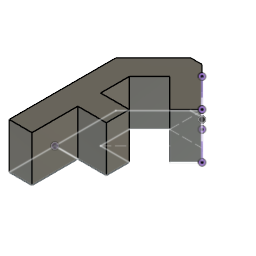
Phototransistor Mount (Autodesk Fusion 360 archive; units mm, degrees)
design "Lab Stand Mount"
Autodesk Fusion 360 part; units mm, degrees
sketch "Sketch1" plane through (0, 0, 0) normal (0, 0, 1) x (1, 0, 0) in component "Lab Stand Mount"
  line L0 (22.5, 0) -> (22.5, 10)
  line L1 (10, 0) -> (10, -20)
  line L2 (22.5, 10) -> (10, 10)
  line L3 (10, 22.5) -> (18.8388, 31.3388)
  line L4 (0, -20) -> (0, 0)
  line L5 (0, 0) -> (22.5, 0)
  line L6 (38.4099, 25.9099) -> (18.8388, 45.481)
  line L7 (10, 10) -> (10, 22.5)
  line L8 (0, 0) -> (10, 0)
  line L9 (31.3388, 18.8388) -> (38.4099, 25.9099)
  line L10 (18.8388, 31.3388) -> (32.981, 31.3388) construction
  line L11 (18.8388, 31.3388) -> (31.3388, 18.8388)
  line L12 (10, 10) -> (25.0888, 25.0888) construction
  line L13 (10, -20) -> (0, -20)
  line L14 (18.8388, 31.3388) -> (18.8388, 45.481) construction
  line L15 (18.8388, 45.481) -> (0, 26.6421)
  line L16 (0, 26.6421) -> (0, 0)
  line L17 (21.3388, 42.981) -> (16.3388, 42.981)
  dimension "d18" = 22.5
  dimension "d19" = 10
  dimension "d20" = 12.5
  dimension "d21" = 12.5
  dimension "d22" = 45
  dimension "d23" = 12.5
  dimension "d24" = 45
  dimension "d25" = 10
  dimension "d28" = 10
  dimension "d29" = 20
  dimension "d43" = 2.5
  constraint coincident L4.end L5.start
  constraint horizontal L5
  constraint perpendicular L0 L5
  constraint perpendicular L0 L2
  constraint perpendicular L2 L7
  constraint horizontal L10
  constraint midpoint L12.end L11
  constraint perpendicular L9 L11
  constraint perpendicular L6 L9
  constraint parallel L3 L12
  constraint horizontal L8
  constraint vertical L1
  constraint horizontal L13
  constraint vertical L4
  constraint perpendicular L10 L14
  constraint coincident L6.end L14
  constraint perpendicular L5 L16
  constraint coincident L6 L17.start
  constraint coincident L15 L17.end
  constraint perpendicular L14 L17
  constraint parallel L3 L15
  constraint coincident L10.end L6
  measures "d18" distance of L4.end L0.start
  measures "d19" distance of L0.end L0.start
  measures "d20" distance of L0.end L2.end
  measures "d21" distance of L2.end L3.start
  measures "d22" angle of L10 L11
  measures "d23" distance of L0.end L11
  measures "d24" angle of L2 L12
  measures "d25" distance of L6.start L9.start
  measures "d28" distance of L4.end L1.start
  measures "d29" distance of L4.start L4.end
  measures "d43" distance of L6.end L17
extrude "Extrude1" add sketch "Sketch1" along normal blind 20 contours L0 L2 L3 L5 L6 L7 L8 L9 L11 L15 L16 L17 | L1 L4 L5 L8 L13 in component "Lab Stand Mount"
sketch "Sketch2" plane through (32.1599, 32.1599, 0) normal (0.707107, 0.707107, 0) x (-0.707107, 0.707107, 0) in component "Lab Stand Mount"
  line L0 (0, 20) -> (0, 0) construction
  line L1 (8.8388, 10) -> (-8.8388, 10) construction
  line L2 (-3.25, 15.6292) -> (-6.5, 10)
  line L3 (-6.5, 10) -> (-3.25, 4.3708)
  line L4 (-3.25, 4.3708) -> (3.25, 4.3708)
  line L5 (3.25, 4.3708) -> (6.5, 10)
  line L6 (6.5, 10) -> (3.25, 15.6292)
  line L7 (3.25, 15.6292) -> (-3.25, 15.6292)
  circle A0 centre (0, 10) radius 3.429
  line L8 (8.8388, 0) -> (-8.8388, 0)
  line L9 (-8.8388, 0) -> (-8.8388, 20)
  line L10 (-8.8388, 20) -> (8.8388, 20)
  line L11 (8.8388, 20) -> (8.8388, 0)
  point P0 (0, 10)
  dimension "d32" = 6.5
  dimension "d38" = 6.858
  constraint coincident L0 P0
  constraint coincident L1 P0
  constraint horizontal L7
  constraint coincident P0 A0.centre
  constraint midpoint L0.start L10
  constraint midpoint L0.end L8
  constraint midpoint L1.end L9
  constraint midpoint L1.start L11
  measures "d32" distance of L2.start L6.end
  measures "d38" diameter of A0
extrude "Extrude2" cut sketch "Sketch2" along normal blind 4.6 from surface at -10 contours L2 L3 L4 L5 L6 L7 | A0 in component "Lab Stand Mount"
extrude "Extrude3" cut sketch "Sketch2" against normal up to surface (10 mm away) contours A0 in component "Lab Stand Mount"
component "Lab Stand Mount" placed x (1, 0, 0) y (0, 1, 0) z (0, 0, 1) at (0, 0, 0)
equation "d18 = d21 + d25"
equation "d20 = d21"
equation "d23 = d21"
equation "d28 = d25"
